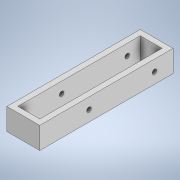
# Autodesk Inventor part: top
Saved by Autodesk Inventor 2022 (Build 260153000, 153)
## iProperties
Created: 2022-11-09
Part Number: top
Material: Generic
Document SubType Name: Modeling
Designer: matys
Density: 1 g/cm^3
Appearance: Default
Author: matys
Autodesk Inventor part; units mm, degrees
ref_plane "YZ Plane" through (0, 0, 0) normal (1, 0, 0) x (0, 1, 0)
ref_plane "XZ Plane" through (0, 0, 0) normal (0, 1, 0) x (-1, 0, 0)
ref_plane "XY Plane" through (0, 0, 0) normal (0, 0, 1) x (1, 0, 0)
sketch "Sketch1" plane through (0, 0, 0) normal (0, 1, 0) x (-1, 0, 0)
  line L0 (0, 0) -> (0, -60)
  line L1 (0, -60) -> (15, -60)
  line L2 (15, -60) -> (15, 0)
  line L3 (15, 0) -> (0, 0)
  line L4 (7.5, -60) -> (12.5, -60)
  line L5 (12.5, -60) -> (12.5, 0)
  line L6 (7.5, -60) -> (2.5, -60)
  line L7 (2.5, -60) -> (2.5, 0)
  line L8 (12.5, 0) -> (12.5, -2.5)
  line L9 (12.5, -2.5) -> (2.5, -2.5)
  line L10 (12.5, -60) -> (12.5, -57.5)
  line L11 (12.5, -57.5) -> (2.5, -57.5)
  line L12 (15, -60) -> (15, -61)
  line L13 (15, -61) -> (0, -61)
  line L14 (0, -61) -> (0, -60)
  line L15 (12.5, -57.5) -> (12.5, -58.5)
  line L16 (12.5, -58.5) -> (2.5, -58.5)
  dimension "d0" = 60
  dimension "d1" = 15
  dimension "d2" = 5
  dimension "d3" = 5
  dimension "d4" = 2.5
  dimension "d5" = 2.5
  dimension "d12" = 1
  dimension "d13" = 1
  constraints: 34 end point, 10 perpendicular, 10 point on line, 2 vertical, 1 midpoint
  measures "d0" distance of L0.start L0.end
  measures "d1" distance of L0.end L1.end
  measures "d2" distance of L4.start L4.end
  measures "d3" distance of L4.start L6.end
  measures "d4" distance of L5.end L8.end
  measures "d5" distance of L4.end L10.end
  measures "d12" distance of L1.end L12.end
  measures "d13" distance of L10.end L15.end
extrude "Extrusion1" add sketch "Sketch1" along normal blind 10 contours L3 L7 L1 L0 | L1 L12 L13 L14 | L3 L5 L9 L7 | L7 L16 L5 L1 | L3 L2 L1 L5
sketch "Sketch2" plane through (0, 0, 0) normal (1, 0, 0) x (0, 0, -1)
  line L0 (61, 10) -> (0, 10) projected
  line L1 (57.5, 0) -> (57.5, 10) projected
  line L2 (60, 10) -> (57.5, 10)
  line L3 (57.5, 10) -> (57.5, 0)
  line L4 (57.5, 0) -> (47.5, 0)
  line L5 (2.5, 0) -> (58.5, 0) projected
  line L6 (47.5, 0) -> (47.5, 10)
  line L7 (2.5, 10) -> (58.5, 10) projected
  line L8 (47.5, 10) -> (57.5, 10)
  line L9 (47.5, 0) -> (57.5, 10)
  line L10 (47.5, 10) -> (57.5, 0)
  circle A0 centre (52.5, 5) radius 1.05
  line L11 (61, 10) -> (60, 10)
  line L12 (60, 10) -> (57.5, 10)
  line L13 (52.5, 5) -> (0, 5)
  line L14 (0, 0) -> (0, 10) projected
  line L15 (0, 5) -> (2.5, 5)
  line L16 (2.5, 0) -> (2.5, 10) projected
  line L17 (2.5, 5) -> (22.5, 5)
  circle A1 centre (22.5, 5) radius 1.05
  dimension "d8" = 10
  dimension "d9" = 2.1
  dimension "d14" = 20
  dimension "d15" = 2.1
  constraints: 24 end point, 4 perpendicular, 3 midpoint, 3 point on line, 2 centre point, 1 coincident, 1 collinear
  measures "d8" distance of L3.end L4.end
  measures "d9" diameter of A0
  measures "d14" distance of L15.end L17.end
  measures "d15" diameter of A1
extrude "Extrusion2" cut sketch "Sketch2" against normal through all contours A0 L10 L9 | L9 L10 A0 | L10 L13 A0 | A0 L9 L10 | L9 A0 L13 | A1 L13 | L13 A1
body "Solid1"
